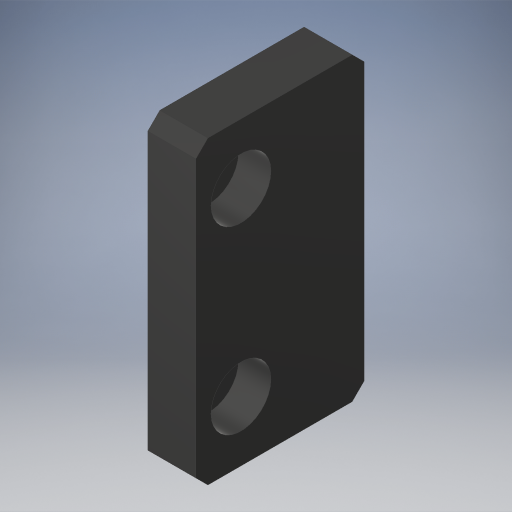
# Autodesk Inventor part: BT503_trajan20_21
Saved by Autodesk Inventor 2023 (Build 270158000, 158)
## iProperties
Company: HTBLA Kaindorf
RuleStatus: InUse
Created: 2022-08-19
Part Number: BT503_trajan20_21
Project: Zeichenmaschine_v2
Material: Kunststoff, undurchsichtig Schwarz
Description: Stifthalter_platte
Document SubType Name: Modeling
Designer: trajan20
Density: 0.952 g/cm^3
Appearance: Glatt - Schwarz
Mass: 9.47245 g
Surface Area: 45.2544 cm^2
Volume: 9.95005 cm^3
AfterDocNew0: iProperties-Editor_aufrufen
Author: jan
Keywords: 2021
Autodesk Inventor part; units mm, degrees
ref_plane "YZ Plane" through (0, 0, 0) normal (1, 0, 0) x (0, 1, 0)
ref_plane "XZ Plane" through (0, 0, 0) normal (0, 1, 0) x (-1, 0, 0)
ref_plane "XY Plane" through (0, 0, 0) normal (0, 0, 1) x (1, 0, 0)
derived "BT501_trajan20_21_Zeichenmaschine_v2_Stifthalter außen.ipt"
sketch "Skizze3" plane through (0, 0, 0) normal (0, 1, 0) x (-1, 0, 0)
  line L0 (0, 0) -> (0, -50)
  line L1 (0, -50) -> (28, -50)
  line L2 (28, -50) -> (28, 0)
  line L3 (28, 0) -> (0, 0)
  point P0 (24, -15)
  point P1 (24, -35)
  point P2 (28, -25)
  point P3 (7.5, -10)
  point P4 (7.5, -40)
  dimension "d4" = 28
  dimension "d5" = 50
  dimension "d6" = 4
  dimension "d7" = 4
  dimension "d8" = 10
  dimension "d9" = 10
  dimension "d10" = 10
  dimension "d11" = 10
  dimension "d12" = 7.5
  dimension "d13" = 7.5
  constraints: 8 end point, 3 perpendicular, 1 midpoint, 1 vertical
  measures "d4" distance between parallel lines of L2 L0
  measures "d5" distance between parallel lines of L3 L1
  measures "d6" distance from line of L2 point (24, -35)
  measures "d7" distance from line of L2 point (24, -15)
  measures "d8" vertical distance of point (28, -25) point (24, -15)
  measures "d9" vertical distance of point (28, -25) point (24, -35)
  measures "d10" distance from line of L1 point (7.5, -40)
  measures "d11" distance from line of L3 point (7.5, -10)
  measures "d12" distance from line of point (7.5, -10) L0
  measures "d13" distance from line of L0 point (7.5, -40)
extrude "Extrusion3" add sketch "Skizze3" along normal blind 8
hole "Bohrung1" at (-24, 0, -35) at (-24, 0, -15) direction (0, 1, 0) diameter 5 depth 6
sketch "Skizze4" plane through (0, 8, 0) normal (0, 1, 0) x (1, 0, 0)
  point P0 (0, 0)
  point P1 (-7.5, 10)
  point P2 (-7.5, 40)
  point P3 (-7.5, 10)
  point P4 (-7.5, 40)
  constraints: 2 coincident
hole "Bohrung2" at (-7.5, 8, -10) at (-7.5, 8, -40) direction (0, -1, 0) diameter 5 end through all counterbore diameter 10 counterbore depth 5.4
chamfer "Fase1" distance 2 angle 45 4 edges at (-28, 4, 0) (0, 4, 0) (0, 4, -50) (-28, 4, -50)
equation "\"d5\" = Haupt_Länge"
equation "\"d6\" = d7"
equation "\"d10\" = d11"
equation "\"d11\" = Federn_Abstand_Breite"
equation "\"d12\" = Federn_Abstand_Länge"
equation "\"d13\" = d12"
equation "\"Haupt_Länge\" = 50"
equation "\"Federn_Abstand_Breite\" = 10"
equation "\"Federn_Abstand_Länge\" = 7.5"
